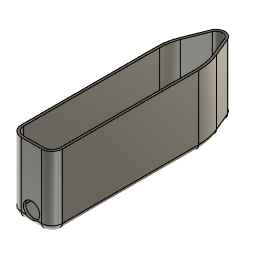
bottom 1-1 (Autodesk Fusion 360 design; units mm, degrees)
Autodesk Fusion 360 part; units mm, degrees
sketch "Sketch1" plane through (0, 0, 0) normal (0, 0, 1) x (1, 0, 0)
  line L0 (-36.1553, -250) -> (-89.3702, -250)
  line L1 (-89.3702, -250) -> (-89.3702, 17.3508)
  line L2 (-89.3702, 17.3508) -> (-36.1553, 17.3508)
  line L3 (-36.1553, 17.3508) -> (-36.1553, -250)
  constraint horizontal L0
  constraint vertical L1
  constraint horizontal L2
  constraint vertical L3
extrude "Extrude1" add sketch "Sketch1" along normal blind 90.7403
sketch "Sketch2" plane through (0, 0, 90.7403) normal (0, 0, 1) x (-1, 0, 0)
  line L0 (36.1553, -17.3508) -> (89.3702, -17.3508)
  line L1 (89.3702, -17.3508) -> (89.3702, 250)
  line L2 (89.3702, 250) -> (36.1553, 250)
  line L3 (36.1553, 250) -> (36.1553, -17.3508)
  line L4 (89.3702, 49.3912) -> (62.7627, -17.3508)
  line L5 (62.7627, -17.3508) -> (36.1553, 46.8639)
  constraint coincident L1 L4.start
  constraint midpoint L0 L4.end
  constraint coincident L3 L5.end
extrude "Extrude2" cut sketch "Sketch2" against normal blind 218.776 contours L0 L3 L5 | L0 L1 L4
fillet "Fillet1" radius 11.437 1 edges at (-62.7627, 17.3508, 45.3701)
fillet "Fillet2" radius 63.498 1 edges at (-89.3702, -49.3912, 45.3701)
fillet "Fillet3" radius 74.946 1 edges at (-36.1553, -46.8639, 45.3701)
fillet "Fillet4" radius 13.769 1 edges at (-89.3702, -250, 45.3701)
fillet "Fillet5" radius 13.342 1 edges at (-36.1553, -250, 45.3701)
shell "Shell1" thickness 3 removed faces 1 at (-53.8936, -178.2217, 90.7403)
fillet "Fillet8" radius 8.009 1 faces at (-53.8936, -178.2217, 0)
hole "Hole2" at (-62.3327, -250, 16.1469) direction (0, 1, 0) diameter 21 depth 30 tip angle 118
